Autodesk Inventor part; units mm, degrees
(part 2 of 2)
sketch "Sketch37" plane through (0, 5.08, 0) normal (0, 1, 0) x (1, 0, 0)
  line L0 (-15.875, 132.715) -> (-5.715, 136.525)
  line L1 (-15.875, 132.715) -> (-5.715, 136.525)
  line L2 (-5.715, 128.905) -> (-5.715, 136.525)
  line L3 (-5.715, 128.905) -> (-5.715, 136.525)
  line L4 (-15.875, 128.905) -> (-15.875, 132.715)
  line L5 (-5.715, 128.905) -> (-5.715, 121.285)
  line L6 (-5.715, 128.905) -> (-5.715, 121.285)
  line L7 (-15.875, 145.7325) -> (-15.875, 112.0775)
  line L8 (-15.875, 145.7325) -> (-15.875, 112.0775)
  line L9 (-15.875, 145.7325) -> (-15.875, 112.0775)
  line L10 (-15.875, 145.7325) -> (-15.875, 112.0775)
  line L11 (-15.875, 110.49) -> (-15.875, 147.32)
  line L12 (-15.875, 73.66) -> (-15.875, 147.32)
  line L13 (-15.875, 128.905) -> (-15.875, 132.715)
  line L14 (-15.875, 128.905) -> (-15.875, 125.095)
  line L15 (-15.875, 128.905) -> (-15.875, 125.095)
  line L16 (-15.875, 125.095) -> (-5.715, 121.285)
  line L17 (-15.875, 125.095) -> (-5.715, 121.285)
  line L18 (-15.875, 73.66) -> (-15.875, 36.83)
  line L19 (-15.875, 90.4875) -> (-15.875, 56.8325)
  line L20 (-15.875, 90.4875) -> (-15.875, 56.8325)
  line L21 (-15.875, 90.4875) -> (-15.875, 56.8325)
  line L22 (-15.875, 90.4875) -> (-15.875, 56.8325)
  line L23 (-15.875, 73.66) -> (-15.875, 69.85)
  line L24 (-15.875, 73.66) -> (-15.875, 69.85)
  line L25 (-5.715, 73.66) -> (-5.715, 66.04)
  line L26 (-15.875, 69.85) -> (-5.715, 66.04)
  line L27 (-15.875, 69.85) -> (-5.715, 66.04)
  line L28 (-5.715, 73.66) -> (-5.715, 66.04)
  line L29 (-15.875, 110.49) -> (-15.875, 73.66)
  line L30 (-15.875, 77.47) -> (-5.715, 81.28)
  line L31 (-5.715, 73.66) -> (-5.715, 81.28)
  line L32 (-15.875, 73.66) -> (-15.875, 77.47)
  line L33 (-5.715, 73.66) -> (-5.715, 81.28)
  line L34 (-15.875, 73.66) -> (-15.875, 77.47)
  line L35 (-15.875, 77.47) -> (-5.715, 81.28)
  line L36 (-5.715, 18.415) -> (-5.715, 10.795)
  line L37 (-5.715, 18.415) -> (-5.715, 10.795)
  line L38 (-15.875, 14.605) -> (-5.715, 10.795)
  line L39 (-15.875, 14.605) -> (-5.715, 10.795)
  line L40 (-15.875, 18.415) -> (-15.875, 14.605)
  line L41 (-15.875, 18.415) -> (-15.875, 14.605)
  line L42 (-15.875, 22.225) -> (-5.715, 26.035)
  line L43 (-15.875, 22.225) -> (-5.715, 26.035)
  line L44 (-5.715, 18.415) -> (-5.715, 26.035)
  line L45 (-5.715, 18.415) -> (-5.715, 26.035)
  line L46 (-15.875, 18.415) -> (-15.875, 22.225)
  line L47 (-15.875, 18.415) -> (-15.875, 22.225)
  line L48 (-15.875, 0) -> (-15.875, 152.4)
  line L49 (20.32, 152.4) -> (-15.875, 152.4)
  line L50 (-15.875, 152.4) -> (-15.875, 0)
  line L51 (-15.875, 0) -> (101.6, 0)
  line L52 (-15.875, 0) -> (101.6, 0)
  line L53 (42.8625, 0) -> (-15.875, 0)
  line L54 (42.8625, 0) -> (101.6, 0)
  line L55 (9.6838, 0) -> (5.8738, -10.16)
  line L56 (9.6838, 0) -> (5.8738, -10.16)
  line L57 (13.4938, -10.16) -> (5.8738, -10.16)
  line L58 (13.4938, -10.16) -> (5.8738, -10.16)
  line L59 (13.4938, 0) -> (9.6838, 0)
  line L60 (13.4938, 0) -> (17.3038, 0)
  line L61 (13.4938, 0) -> (17.3038, 0)
  line L62 (17.3038, 0) -> (21.1138, -10.16)
  line L63 (13.4938, -10.16) -> (21.1138, -10.16)
  line L64 (13.4938, -10.16) -> (21.1138, -10.16)
  line L65 (17.3038, 0) -> (21.1138, -10.16)
  line L66 (13.4938, 0) -> (9.6838, 0)
  line L67 (72.2313, 0) -> (68.4213, 0)
  line L68 (72.2313, 0) -> (68.4213, 0)
  line L69 (68.4213, 0) -> (64.6113, -10.16)
  line L70 (72.2313, -10.16) -> (64.6113, -10.16)
  line L71 (72.2313, -10.16) -> (64.6112, -10.16)
  line L72 (68.4213, 0) -> (64.6112, -10.16)
  line L73 (72.2313, 0) -> (76.0413, 0)
  line L74 (72.2313, 0) -> (76.0413, 0)
  line L75 (72.2313, -10.16) -> (79.8513, -10.16)
  line L76 (72.2313, -10.16) -> (79.8513, -10.16)
  line L77 (76.0413, 0) -> (79.8513, -10.16)
  line L78 (76.0413, 0) -> (79.8513, -10.16)
  line L79 (-15.875, 132.715) -> (-5.715, 136.525)
  line L80 (-15.875, 132.715) -> (-5.715, 136.525)
  line L81 (-5.715, 128.905) -> (-5.715, 136.525)
  line L82 (-5.715, 128.905) -> (-5.715, 136.525)
  line L83 (-15.875, 128.905) -> (-15.875, 132.715)
  line L84 (-5.715, 128.905) -> (-5.715, 121.285)
  line L85 (-5.715, 128.905) -> (-5.715, 121.285)
  line L86 (-15.875, 145.7325) -> (-15.875, 112.0775)
  line L87 (-15.875, 145.7325) -> (-15.875, 112.0775)
  line L88 (-15.875, 145.7325) -> (-15.875, 112.0775)
  line L89 (-15.875, 145.7325) -> (-15.875, 112.0775)
  line L90 (-15.875, 110.49) -> (-15.875, 147.32)
  line L91 (-15.875, 73.66) -> (-15.875, 147.32)
  line L92 (-15.875, 128.905) -> (-15.875, 132.715)
  line L93 (-15.875, 128.905) -> (-15.875, 125.095)
  line L94 (-15.875, 128.905) -> (-15.875, 125.095)
  line L95 (-15.875, 125.095) -> (-5.715, 121.285)
  line L96 (-15.875, 125.095) -> (-5.715, 121.285)
  line L97 (-15.875, 73.66) -> (-15.875, 36.83)
  line L98 (-15.875, 90.4875) -> (-15.875, 56.8325)
  line L99 (-15.875, 90.4875) -> (-15.875, 56.8325)
  line L100 (-15.875, 90.4875) -> (-15.875, 56.8325)
  line L101 (-15.875, 90.4875) -> (-15.875, 56.8325)
  line L102 (-15.875, 73.66) -> (-15.875, 69.85)
  line L103 (-15.875, 73.66) -> (-15.875, 69.85)
  line L104 (-5.715, 73.66) -> (-5.715, 66.04)
  line L105 (-15.875, 69.85) -> (-5.715, 66.04)
  line L106 (-15.875, 69.85) -> (-5.715, 66.04)
  line L107 (-5.715, 73.66) -> (-5.715, 66.04)
  line L108 (-15.875, 110.49) -> (-15.875, 73.66)
  line L109 (-15.875, 77.47) -> (-5.715, 81.28)
  line L110 (-5.715, 73.66) -> (-5.715, 81.28)
  line L111 (-15.875, 73.66) -> (-15.875, 77.47)
  line L112 (-5.715, 73.66) -> (-5.715, 81.28)
  line L113 (-15.875, 73.66) -> (-15.875, 77.47)
  line L114 (-15.875, 77.47) -> (-5.715, 81.28)
  line L115 (-5.715, 18.415) -> (-5.715, 10.795)
  line L116 (-5.715, 18.415) -> (-5.715, 10.795)
  line L117 (-15.875, 14.605) -> (-5.715, 10.795)
  line L118 (-15.875, 14.605) -> (-5.715, 10.795)
  line L119 (-15.875, 18.415) -> (-15.875, 14.605)
  line L120 (-15.875, 18.415) -> (-15.875, 14.605)
  line L121 (-15.875, 22.225) -> (-5.715, 26.035)
  line L122 (-15.875, 22.225) -> (-5.715, 26.035)
  line L123 (-5.715, 18.415) -> (-5.715, 26.035)
  line L124 (-5.715, 18.415) -> (-5.715, 26.035)
  line L125 (-15.875, 18.415) -> (-15.875, 22.225)
  line L126 (-15.875, 18.415) -> (-15.875, 22.225)
  line L127 (-15.875, 0) -> (-15.875, 152.4)
  line L128 (20.32, 152.4) -> (-15.875, 152.4)
  line L129 (-15.875, 152.4) -> (-15.875, 0)
  line L130 (-15.875, 0) -> (101.6, 0)
  line L131 (-15.875, 0) -> (101.6, 0)
  line L132 (42.8625, 0) -> (-15.875, 0)
  line L133 (42.8625, 0) -> (101.6, 0)
  line L134 (9.6838, 0) -> (5.8738, -10.16)
  line L135 (9.6838, 0) -> (5.8738, -10.16)
  line L136 (13.4938, -10.16) -> (5.8738, -10.16)
  line L137 (13.4938, -10.16) -> (5.8738, -10.16)
  line L138 (13.4938, 0) -> (9.6838, 0)
  line L139 (13.4938, 0) -> (17.3038, 0)
  line L140 (13.4938, 0) -> (17.3038, 0)
  line L141 (17.3038, 0) -> (21.1138, -10.16)
  line L142 (13.4938, -10.16) -> (21.1138, -10.16)
  line L143 (13.4938, -10.16) -> (21.1138, -10.16)
  line L144 (17.3038, 0) -> (21.1138, -10.16)
  line L145 (13.4938, 0) -> (9.6838, 0)
  line L146 (72.2313, 0) -> (68.4213, 0)
  line L147 (72.2313, 0) -> (68.4213, 0)
  line L148 (68.4213, 0) -> (64.6113, -10.16)
  line L149 (72.2313, -10.16) -> (64.6113, -10.16)
  line L150 (72.2313, -10.16) -> (64.6112, -10.16)
  line L151 (68.4213, 0) -> (64.6112, -10.16)
  line L152 (72.2313, 0) -> (76.0413, 0)
  line L153 (72.2313, 0) -> (76.0413, 0)
  line L154 (72.2313, -10.16) -> (79.8513, -10.16)
  line L155 (72.2313, -10.16) -> (79.8513, -10.16)
  line L156 (76.0413, 0) -> (79.8513, -10.16)
  line L157 (76.0413, 0) -> (79.8513, -10.16)
  point P0 (0, 0)
  point P1 (-15.875, 35.2425)
  point P2 (-15.875, 35.2425)
  point P3 (-15.875, 35.2425)
  point P4 (-15.875, 35.2425)
  constraints: 312 end point, 18 point on line, 12 midpoint, 4 collinear, 4 horizontal, 6 other
extrude "Extrusion34" add sketch "Sketch36" against normal blind 5.08 contours L51 L61 L63 L55 L57 | L51 L74 L75 L69 L67
extrude "Extrusion35" cut sketch "Sketch37" against normal blind 5.08 contours L0 L2 L5 L16 L7 L4 | L12 L30 L31 L25 L26 L18 | L36 L38 L40 L46 L42 L44
body "Solid2"
